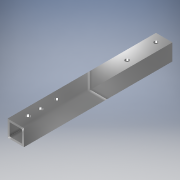
# Autodesk Inventor part: 15102898-16-A-0205
Saved by Autodesk Inventor 2017 (Build 210142000, 142)
## iProperties
Created: 2016-09-30
Part Number: 15102898-16-A-0205
Material: Aluminum 6061
Document SubType Name: Modeling
Designer: gus
Density: 2.7 g/cm^3
Appearance: Aluminum - Flat
Mass: 172.586 g
Surface Area: 412.096 cm^2
Volume: 63.9208 cm^3
Author: gus
Autodesk Inventor part; units mm, degrees
ref_plane "YZ Plane" through (0, 0, 0) normal (1, 0, 0) x (0, 1, 0)
ref_plane "XZ Plane" through (0, 0, 0) normal (0, 1, 0) x (-1, 0, 0)
ref_plane "XY Plane" through (0, 0, 0) normal (0, 0, 1) x (1, 0, 0)
sketch "Sketch1" plane through (0, 0, 0) normal (0, 0, 1) x (1, 0, 0)
  line L0 (0, 0) -> (-25.4, 0)
  line L1 (-25.4, 0) -> (-25.4, -25.4)
  line L2 (-25.4, -25.4) -> (0, -25.4)
  line L3 (0, -25.4) -> (0, 0)
  line L4 (-3.175, -22.225) -> (-22.225, -22.225)
  line L5 (-22.225, -22.225) -> (-22.225, -3.175)
  line L6 (-22.225, -3.175) -> (-3.175, -3.175)
  line L7 (-3.175, -3.175) -> (-3.175, -22.225)
  dimension "d0" = 25.4
  dimension "d1" = 25.4
  dimension "d2" = 3.175
  constraints: 16 end point, 4 parallel, 2 perpendicular, 1 horizontal, 3 other
  measures "d0" distance of L2.end L1.end
  measures "d1" distance of L1.end L0.end
  measures "d2" distance between parallel lines of L2 L4
extrude "Extrusion1" add sketch "Sketch1" along normal blind 228.6
sketch "Sketch2" plane through (-25.4, -25.4, 0) normal (0, -1, 0) x (1, 0, 0)
  circle A0 centre (12.7, 190.5) radius 3.175
  line L0 (0, 228.6) -> (25.4, 228.6) projected
  line L1 (0, 0) -> (0, 228.6) projected
  circle A1 centre (12.7, 12.7) radius 3.175
  circle A2 centre (14.2875, 58.7375) radius 3.175
  line L2 (0, 0) -> (25.4, 0) projected
  circle A3 centre (12.7, 209.55) radius 3.3734
  line L3 (25.4, 0) -> (25.4, 228.6) projected
  circle A4 centre (12.7, 165.1) radius 3.175
  dimension "d5" = 6.35
  dimension "d6" = 38.1
  dimension "d7" = 12.7
  dimension "d10" = 6.35
  dimension "d11" = 12.7
  dimension "d13" = 14.2875
  dimension "d14" = 12.7
  dimension "d15" = 58.7375
  dimension "d16" = 6.7469
  dimension "d17" = 12.7
  dimension "d18" = 19.05
  dimension "d19" = 6.35
  dimension "d20" = 63.5
  dimension "d21" = 12.7
  constraints: 5 centre point, 1 equal radius
  measures "d5" diameter of A0
  measures "d6" distance from line of L0 A0.centre
  measures "d7" distance from line of L1 A0.centre
  measures "d10" diameter of A2
  measures "d11" distance from line of L2 A1.centre
  measures "d13" distance from line of L1 A2.centre
  measures "d14" distance from line of L1 A1.centre
  measures "d15" distance from line of L2 A2.centre
  measures "d16" diameter of A3
  measures "d17" distance from line of L3 A3.centre
  measures "d18" distance from line of A3.centre L0
  measures "d19" diameter of A4
  measures "d20" distance from line of L0 A4.centre
  measures "d21" distance from line of L1 A4.centre
extrude "Extrusion2" cut sketch "Sketch2" against normal blind 152.4 contours A0 | A1 | A2 | A3 | A4
body "Solid1"
